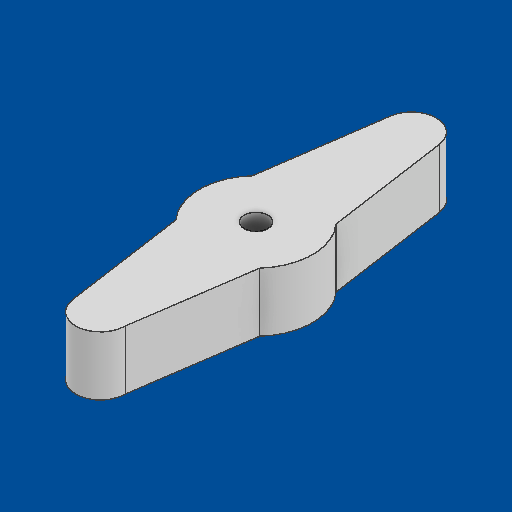
# Autodesk Inventor part: servo_attach
Saved by Autodesk Inventor 2026.2 (Build 302298000, 298)
## iProperties
Created: 2026-02-24
Part Number: servo_attach
Material: Generic
Document SubType Name: Modeling
Designer: Thoma
Density: 1 g/cm^3
Appearance: Default
Author: Thoma
Autodesk Inventor part; units mm, degrees
ref_plane "YZ Plane" through (0, 0, 0) normal (1, 0, 0) x (0, 1, 0)
ref_plane "XZ Plane" through (0, 0, 0) normal (0, 1, 0) x (-1, 0, 0)
ref_plane "XY Plane" through (0, 0, 0) normal (0, 0, 1) x (1, 0, 0)
sketch "Sketch1" plane through (0, 0, 0) normal (0, 1, 0) x (-1, 0, 0)
  circle A0 centre (0, 0) radius 5.95
  circle A1 centre (0, -16.35) radius 2.6
  line L0 (4.4, -4.0053) -> (2.5736, -16.7197)
  circle A2 centre (0, 16.35) radius 2.6
  line L1 (4.4, 4.0053) -> (2.5736, 16.7197)
  line L2 (-4.4, 4.0053) -> (-2.6, 16.35)
  line L3 (-4.4, -4.0053) -> (-2.5736, -16.7197)
  dimension "d0" = 11.9
  dimension "d1" = 5.2
  dimension "d2" = 4.4
  dimension "d3" = 5.2
  dimension "d4" = 16.35
  dimension "d5" = 16.35
  dimension "d6" = 4.4
  dimension "d7" = 4.4
  dimension "d8" = 4.4
  dimension "d9" = 0
  constraints: 8 end point, 8 point on circle, 3 centre point, 3 tangent, 1 coincident
  measures "d0" diameter of A0
  measures "d1" diameter of A1
  measures "d2" horizontal distance of point (0, 0) L0.start
  measures "d3" diameter of A2
  measures "d4" distance of point (0, 0) A2.centre
  measures "d5" distance of A1.centre point (0, 0)
  measures "d6" horizontal distance of point (0, 0) L1.start
  measures "d7" horizontal distance of point (0, 0) L2.start
  measures "d8" horizontal distance of point (0, 0) L3.start
  measures "d9" horizontal distance of point (0, 0) A1.centre
extrude "Extrusion1" add sketch "Sketch1" along normal blind 2.2
sketch "Sketch2" plane through (0, 0, 0) normal (0, -1, 0) x (1, 0, 0)
  circle A0 centre (0, 0) radius 3.8734
  circle A1 centre (0, 0) radius 3.45
  dimension "d12" = 6.9
  constraints: 2 centre point, 2 coincident
  measures "d12" diameter of A1
extrude "Extrusion2" add sketch "Sketch2" along normal blind 3.2
sketch "Sketch3" plane through (0, 2.2, 0) normal (0, 1, 0) x (1, 0, 0)
  circle A0 centre (0, 0) radius 1.25
  dimension "d15" = 2.5
  constraints: 1 centre point, 1 coincident
  measures "d15" diameter of A0
extrude "Extrusion3" cut sketch "Sketch3" against normal blind 2.2
thicken "Thicken1" operation add thickness 4 both sides no extend neighbours no toward (0, -1, 0) faces at (0.1556, 0, -12.4282)
body "Solid1"
